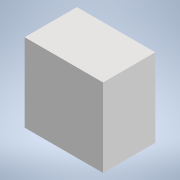
# Autodesk Inventor part: Holder Base
Saved by Autodesk Inventor 2022 (Build 260153000, 153)
## iProperties
Created: 2022-03-02
Part Number: Holder Base
Material: Generic
Document SubType Name: Modeling
Designer: Nathan Griffith
Density: 1 g/cm^3
Appearance: Default
Author: Nathan Griffith
Autodesk Inventor part; units mm, degrees
ref_plane "YZ Plane" through (0, 0, 0) normal (1, 0, 0) x (0, 1, 0)
ref_plane "XZ Plane" through (0, 0, 0) normal (0, 1, 0) x (-1, 0, 0)
ref_plane "XY Plane" through (0, 0, 0) normal (0, 0, 1) x (1, 0, 0)
sketch "Sketch1" plane through (0, 0, 0) normal (0, 0, 1) x (1, 0, 0)
  line L0 (38.1, 38.1) -> (-38.1, 38.1)
  line L1 (-38.1, 38.1) -> (-38.1, -38.1)
  line L2 (-38.1, -38.1) -> (38.1, -38.1)
  line L3 (38.1, -38.1) -> (38.1, 38.1)
  line L4 (38.1, 38.1) -> (-38.1, -38.1) construction
  line L5 (-38.1, 38.1) -> (38.1, -38.1) construction
  line L6 (35.052, 35.052) -> (-35.052, 35.052) construction
  line L7 (-35.052, 35.052) -> (-35.052, -35.052) construction
  line L8 (-35.052, -35.052) -> (35.052, -35.052) construction
  line L9 (35.052, -35.052) -> (35.052, 35.052) construction
  line L10 (35.052, 35.052) -> (-35.052, -35.052) construction
  line L11 (-35.052, 35.052) -> (35.052, -35.052) construction
  line L12 (-35.052, -35.052) -> (-15.24, -35.052)
  line L13 (-15.24, -35.052) -> (-15.24, -15.24)
  line L14 (-15.24, -15.24) -> (-35.052, -15.24)
  line L15 (-35.052, -15.24) -> (-35.052, -35.052)
  line L16 (-9.652, -35.052) -> (10.16, -35.052)
  line L17 (10.16, -35.052) -> (10.16, -15.24)
  line L18 (10.16, -15.24) -> (-9.652, -15.24)
  line L19 (-9.652, -15.24) -> (-9.652, -35.052)
  line L20 (15.748, -35.052) -> (35.56, -35.052)
  line L21 (35.56, -35.052) -> (35.56, -15.24)
  line L22 (35.56, -15.24) -> (15.748, -15.24)
  line L23 (15.748, -15.24) -> (15.748, -35.052)
  line L24 (-15.24, 10.16) -> (-35.052, 10.16)
  line L25 (-35.052, 10.16) -> (-35.052, -9.652)
  line L26 (-15.24, -9.652) -> (-15.24, 10.16)
  line L27 (-9.652, 10.16) -> (-9.652, -9.652)
  line L28 (10.16, 10.16) -> (-9.652, 10.16)
  line L29 (10.16, -9.652) -> (10.16, 10.16)
  line L30 (15.748, 10.16) -> (15.748, -9.652)
  line L31 (35.56, 10.16) -> (15.748, 10.16)
  line L32 (35.56, -9.652) -> (35.56, 10.16)
  line L33 (15.748, -9.652) -> (35.56, -9.652)
  line L34 (-9.652, -9.652) -> (10.16, -9.652)
  line L35 (-15.24, 35.56) -> (-35.052, 35.56)
  line L36 (-35.052, 35.56) -> (-35.052, 15.748)
  line L37 (-15.24, 15.748) -> (-15.24, 35.56)
  line L38 (-9.652, 35.56) -> (-9.652, 15.748)
  line L39 (10.16, 35.56) -> (-9.652, 35.56)
  line L40 (10.16, 15.748) -> (10.16, 35.56)
  line L41 (15.748, 35.56) -> (15.748, 15.748)
  line L42 (35.56, 35.56) -> (15.748, 35.56)
  line L43 (35.56, 15.748) -> (35.56, 35.56)
  line L44 (15.748, 15.748) -> (35.56, 15.748)
  line L45 (-9.652, 15.748) -> (10.16, 15.748)
  line L46 (-35.052, -9.652) -> (-15.24, -9.652)
  line L47 (-35.052, 15.748) -> (-15.24, 15.748)
  point P0 (0, 0)
  dimension "d0" = 76.2
  dimension "d1" = 76.2
  dimension "d2" = 70.104
  dimension "d3" = 19.812
  dimension "d4" = 19.812
  dimension "d7" = 25.4
  dimension "d14" = 25.4
  constraints: 96 end point, 7 parallel, 5 horizontal, 4 midpoint, 3 perpendicular, 2 point on line, 1 vertical, 62 other
  measures "d0" distance of L2.end L1.end
  measures "d1" distance of L1.end L0.end
  measures "d2" distance of L8.end L7.end
  measures "d3" distance of L14.end L13.end
  measures "d4" distance of L13.end L12.end
  measures "d7" distance of L7.end L16.start
  measures "d14" distance of L13.end L24.start
extrude "Extrusion1" add sketch "Sketch1" against normal blind 10.668
sketch "Sketch2" plane through (0, 0, 0) normal (0, 0, 1) x (1, 0, 0)
  line L0 (-38.1, 38.1) -> (-38.1, -38.1) projected
  line L1 (-38.1, -38.1) -> (38.1, -38.1) projected
  line L2 (38.1, -38.1) -> (38.1, 38.1) projected
  line L3 (38.1, 38.1) -> (-38.1, 38.1) projected
  line L4 (15.748, 35.56) -> (35.56, 35.56) projected
  line L5 (35.56, 35.56) -> (35.56, 15.748) projected
  line L6 (35.56, 15.748) -> (15.748, 15.748) projected
  line L7 (15.748, 15.748) -> (15.748, 35.56) projected
  line L8 (-9.652, 35.56) -> (10.16, 35.56) projected
  line L9 (10.16, 35.56) -> (10.16, 15.748) projected
  line L10 (10.16, 15.748) -> (-9.652, 15.748) projected
  line L11 (-9.652, 15.748) -> (-9.652, 35.56) projected
  line L12 (-15.24, 35.56) -> (-15.24, 15.748) projected
  line L13 (-15.24, 15.748) -> (-35.052, 15.748) projected
  line L14 (-35.052, 15.748) -> (-35.052, 35.56) projected
  line L15 (-35.052, 35.56) -> (-15.24, 35.56) projected
  line L16 (15.748, 10.16) -> (35.56, 10.16) projected
  line L17 (35.56, 10.16) -> (35.56, -9.652) projected
  line L18 (35.56, -9.652) -> (15.748, -9.652) projected
  line L19 (15.748, -9.652) -> (15.748, 10.16) projected
  line L20 (-9.652, 10.16) -> (10.16, 10.16) projected
  line L21 (10.16, 10.16) -> (10.16, -9.652) projected
  line L22 (10.16, -9.652) -> (-9.652, -9.652) projected
  line L23 (-9.652, -9.652) -> (-9.652, 10.16) projected
  line L24 (-15.24, 10.16) -> (-15.24, -9.652) projected
  line L25 (-15.24, -9.652) -> (-35.052, -9.652) projected
  line L26 (-35.052, -9.652) -> (-35.052, 10.16) projected
  line L27 (-35.052, 10.16) -> (-15.24, 10.16) projected
  line L28 (15.748, -35.052) -> (15.748, -15.24) projected
  line L29 (15.748, -15.24) -> (35.56, -15.24) projected
  line L30 (35.56, -15.24) -> (35.56, -35.052) projected
  line L31 (35.56, -35.052) -> (15.748, -35.052) projected
  line L32 (-9.652, -35.052) -> (-9.652, -15.24) projected
  line L33 (-9.652, -15.24) -> (10.16, -15.24) projected
  line L34 (10.16, -15.24) -> (10.16, -35.052) projected
  line L35 (10.16, -35.052) -> (-9.652, -35.052) projected
  line L36 (-35.052, -35.052) -> (-35.052, -15.24) projected
  line L37 (-35.052, -15.24) -> (-15.24, -15.24) projected
  line L38 (-15.24, -15.24) -> (-15.24, -35.052) projected
  line L39 (-15.24, -35.052) -> (-35.052, -35.052) projected
  line L40 (38.1, 38.1) -> (-38.1, 38.1)
  line L41 (-38.1, 38.1) -> (-38.1, -38.1)
  line L42 (-38.1, -38.1) -> (38.1, -38.1)
  line L43 (38.1, -38.1) -> (38.1, 38.1)
  point P0 (0, 0)
  constraints: 8 end point, 2 parallel, 1 horizontal, 1 perpendicular
extrude "Extrusion2" add sketch "Sketch2" along normal blind 40.132 contours L3 L2 L1 L0 | L4 L5 L6 L7 | L8 L9 L10 L11 | L12 L13 L14 L15 | L16 L17 L18 L19 | L20 L21 L22 L23 | L24 L25 L26 L27 | L28 L29 L30 L31 | L32 L33 L34 L35 | L36 L37 L38 L39
body "Solid1"
